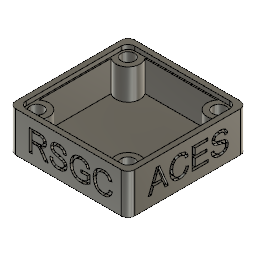
MyLEDTesterCase (Autodesk Fusion 360 design; units mm, degrees)
Autodesk Fusion 360 part; units mm, degrees
note: some values were not read from the file. Chosen so that the rebuilt part matches the saved one: that a step has no effect; the layout of a text. Set by a fixed rule: which sketch regions a step uses.
sketch "PCB" plane through (0, 0, 0) normal (0, 0, 1) x (1, 0, 0)
  line L0 (0, 0) -> (40, 0)
  line L1 (40, 0) -> (40, 40)
  line L2 (40, 40) -> (0, 40)
  line L3 (0, 40) -> (0, 0)
  line L4 (-0.25, -0.25) -> (40.25, -0.25)
  line L5 (40.25, -0.25) -> (40.25, 40.25)
  line L6 (40.25, 40.25) -> (-0.25, 40.25)
  line L7 (-0.25, 40.25) -> (-0.25, -0.25)
  line L8 (39.75, 0.25) -> (39.75, 39.75)
  line L9 (39.75, 39.75) -> (0.25, 39.75)
  line L10 (0.25, 39.75) -> (0.25, 0.25)
  line L11 (0.25, 0.25) -> (39.75, 0.25)
  line L12 (42.25, 42.25) -> (-2.25, 42.25)
  line L13 (-2.25, 42.25) -> (-2.25, -2.25)
  line L14 (-2.25, -2.25) -> (42.25, -2.25)
  line L15 (42.25, -2.25) -> (42.25, 42.25)
  dimension "d7" = 40
  dimension "d8" = 40
  dimension "d30" = 0.25
  dimension "d32" = 2.25
  constraint horizontal L0
  constraint vertical L1
  constraint horizontal L2
  constraint vertical L3
  constraint coincident L0.start L3.end
  measures "d7" distance of L0.start L0.end
  measures "d8" distance of L0.start L2.end
sketch "Piers" plane through (0, 0, 0) normal (0, 0, 1) x (1, 0, 0)
  line L0 (40, 40) -> (0, 40)
  circle A0 centre (3, 37) radius 4.5
  circle A1 centre (3, 37) radius 2.5
  line L1 (0, 40) -> (0, 0)
  line L2 (0, 0) -> (40, 0)
  circle A2 centre (3, 3) radius 4.5
  circle A3 centre (3, 3) radius 2.5
  line L3 (40, 0) -> (40, 40)
  circle A4 centre (37, 37) radius 4.5
  circle A5 centre (37, 37) radius 2.5
  circle A6 centre (37, 3) radius 4.5
  circle A7 centre (37, 3) radius 2.5
  point P0 (3, 37)
  point P1 (0, 40)
  point P2 (3, 3)
  point P3 (37, 37)
  point P4 (37, 3)
  point P5 (37, 3)
  dimension "d10" = 3
  dimension "d11" = 3
  dimension "d13" = 9
  dimension "d15" = 5
  dimension "d16" = 3
  dimension "d17" = 3
  dimension "d18" = 9
  dimension "d19" = 5
  dimension "d20" = 3
  dimension "d21" = 3
  dimension "d22" = 9
  dimension "d23" = 5
  dimension "d24" = 3
  dimension "d25" = 3
  dimension "d26" = 9
  dimension "d27" = 5
  constraint coincident P0 A0.centre
  constraint coincident P2 A2.centre
  constraint coincident P3 A4.centre
  constraint coincident P5 P4
  constraint concentric A6 A7
  measures "d10" horizontal distance of P0 L0.end
  measures "d11" distance of P0 L0
  measures "d13" diameter of A0
  measures "d15" diameter of A1
  measures "d16" distance of P2 L1
  measures "d17" distance of P2 L2
  measures "d18" diameter of A2
  measures "d19" diameter of A3
  measures "d20" distance of P3 L3
  measures "d21" distance of L0 P3
  measures "d22" diameter of A4
  measures "d23" diameter of A5
  measures "d24" distance of L3 P5
  measures "d25" distance of L2 P5
  measures "d26" diameter of A6
  measures "d27" diameter of A7
extrude "Extrude1" add sketch "Piers" along normal blind 13.4 contours L0 L3 A4 | L0 L3 A4 makes body 1
extrude "Extrude2" add sketch "Piers" along normal blind 6 contours A5 bodies 1
extrude "Extrude3" add sketch "Piers" along normal blind 6 separate body contours A7 makes body 2
extrude "Extrude4" add sketch "Piers" along normal blind 13.4 contours L2 L3 A6 | L2 L3 A6 bodies 2
extrude "Extrude5" add sketch "Piers" along normal blind 6 separate body contours A3 makes body 3
extrude "Extrude6" add sketch "Piers" along normal blind 13.4 contours L1 L2 A2 | L1 L2 A2 bodies 3
extrude "Extrude7" add sketch "Piers" along normal blind 6 separate body contours A1 makes body 4
extrude "Extrude8" add sketch "Piers" along normal blind 13.4 contours L0 A0 L1 | L0 A0 L1 bodies 4
extrude "Extrude9" cut sketch "PCB" along normal blind 2 contours L8 L9 L10 L11 bodies 1 2 3 4
extrude "Extrude10" add sketch "PCB" along normal blind 2 contours L8 L9 L10 L11 bodies 1 2 3 4
extrude "Extrude11" add sketch "PCB" along normal blind 13.4 contours L0 L1 L2 L3 bodies 1
extrude "Extrude12" add sketch "PCB" along normal blind 13.4 contours L4 L5 L6 L7 bodies 1
extrude "Extrude13" add sketch "PCB" along normal blind 15 contours L12 L13 L14 L15 bodies 1
fillet "Fillet1" radius 2.54 4 edges at (42.25, -2.25, 7.5) (-2.25, -2.25, 7.5) (42.25, 42.25, 7.5) (-2.25, 42.25, 7.5) on bodies 1
fillet "Fillet2" radius 2.54 1 edges at (40.25, -0.25, 14.2) on bodies 1
fillet "Fillet3" radius 2.54 1 edges at (-0.25, 40.25, 14.2) on bodies 1
fillet "Fillet4" radius 2.54 1 edges at (-0.25, -0.25, 14.2) on bodies 1
fillet "Fillet5" radius 2.54 1 edges at (40.25, 40.25, 14.2) on bodies 1
extrude "Extrude15" [no effect]
sketch "Sketch14" plane through (0, -2.25, 0) normal (0, -1, 0) x (1, 0, 0)
  line L0 (0.29, 15) -> (0.29, 0)
  line L1 (0.29, 0) -> (39.71, 0)
  line L2 (39.71, 0) -> (39.71, 15)
  line L3 (39.71, 15) -> (0.29, 15)
  line L4 (3.6628, 2.2796) -> (38.1217, 2.2796) construction
  line L5 (38.1217, 2.2796) -> (38.1217, 12.6948) construction
  line L6 (38.1217, 12.6948) -> (3.6628, 12.6948) construction
  line L7 (3.6628, 12.6948) -> (3.6628, 2.2796) construction
  line L8 (20, 15) -> (20, 0) construction
  line L9 (0.29, 7.5) -> (39.71, 7.5) construction
  dimension "d84" = 8
  text T0 "RSGC" font "Arial" height 8 align centre middle in box 34.4588 x 10.4152 at (3.6628, 2.2796) x (1, 0) y (0, 1) spacing 1
  constraint midpoint L3 L8.start
  constraint midpoint L1 L8.end
  constraint midpoint L0 L9.start
  constraint midpoint L2 L9.end
extrude "Extrude16" cut sketch "Sketch14" against normal blind 1 text T0 bodies 1
sketch "Sketch15" plane through (42.25, 0, 0) normal (1, 0, 0) x (0, 1, 0)
  line L0 (39.71, 0) -> (39.71, 15)
  line L1 (39.71, 15) -> (0.29, 15)
  line L2 (0.29, 15) -> (0.29, 0)
  line L3 (0.29, 0) -> (39.71, 0)
  line L4 (2.6602, 2.4104) -> (37.8312, 2.4104) construction
  line L5 (37.8312, 2.4104) -> (37.8312, 13.0108) construction
  line L6 (37.8312, 13.0108) -> (2.6602, 13.0108) construction
  line L7 (2.6602, 13.0108) -> (2.6602, 2.4104) construction
  dimension "d87" = 8
  text T0 "ACES" font "Arial" height 8 align centre middle in box 35.171 x 10.6004 at (2.6602, 2.4104) x (1, 0) y (0, 1) spacing 1
extrude "Extrude17" cut sketch "Sketch15" against normal blind 1 text T0 bodies 1
sketch "Sketch16" plane through (0, 42.25, 0) normal (0, 1, 0) x (-1, 0, 0)
  line L0 (-0.29, 0) -> (-0.29, 15)
  line L1 (-0.29, 15) -> (-39.71, 15)
  line L2 (-39.71, 15) -> (-39.71, 0)
  line L3 (-39.71, 0) -> (-0.29, 0)
  line L4 (-38.4676, 1.9614) -> (-1.8104, 1.9614) construction
  line L5 (-1.8104, 1.9614) -> (-1.8104, 13.8308) construction
  line L6 (-1.8104, 13.8308) -> (-38.4676, 13.8308) construction
  line L7 (-38.4676, 13.8308) -> (-38.4676, 1.9614) construction
  dimension "d90" = 4
  text T0 "LED Tester" font "Arial" height 4 align centre middle in box 36.6572 x 11.8695 at (-38.4676, 1.9614) x (1, 0) y (0, 1) spacing 1 kerned
extrude "Extrude18" cut sketch "Sketch16" against normal blind 1 text T0 bodies 1
sketch "Revised_ACESLogoOutline-01" plane through (-2.25, 14.4902, 3.4358) normal (-1, 0, 0) x (0, -1, 0)
  line L0 (5.7875, 4.2153) -> (5.7875, 5.4361)
  spline S0 degree 3 poles (5.7875, 5.4361) (5.7875, 5.4722) (5.7722, 5.5181) (5.8194, 5.5347) knots 1 1 1 1 2 2 2 2
  arc A0 (5.8194, 5.5347) -> (5.9472, 5.5069) centre (5.8593, 5.4104) cw
  arc A1 (5.9472, 5.5069) -> (6.075, 5.3583) centre (5.2544, 4.782) cw
  spline S1 degree 3 poles (6.075, 5.3583) (6.3458, 5.0319) (6.6208, 4.7069) (6.8833, 4.3736) knots 4 4 4 4 5 5 5 5
  spline S2 degree 3 poles (6.8833, 4.3736) (7.1224, 4.1027) (7.0966, 3.6893) (6.8257, 3.4503) (6.6775, 3.3195) (6.4782, 3.2628) (6.2833, 3.2958) knots 5 5 5 5 6 6 6 7 7 7 7
  spline S3 degree 3 poles (6.2833, 3.2958) (6.2083, 3.3069) (6.1361, 3.3194) (6.0625, 3.3375) knots 7 7 7 7 8 8 8 8
  spline S4 degree 3 poles (6.0625, 3.3375) (6.0514, 3.3375) (6.0417, 3.3528) (6.0194, 3.3222) (6.0306, 3.3167) (6.0306, 3.3042) knots 8 8 8 8 9 9 10 10 10 10
  arc A2 (6.0306, 3.3042) -> (6.1597, 3.0264) centre (7.2606, 3.7072) ccw
  spline S5 degree 3 poles (6.1597, 3.0264) (6.1819, 2.9875) (6.2264, 2.9514) (6.1736, 2.8542) (6.1181, 2.875) (6.075, 2.8736) knots 11 11 11 11 12 12 13 13 13 13
  line L1 (6.075, 2.8736) -> (5.8667, 2.8736)
  spline S6 degree 3 poles (5.8667, 2.8736) (5.7972, 2.8736) (5.7861, 2.8875) (5.7861, 2.9528) knots 14 14 14 14 15 15 15 15
  line L2 (5.7861, 2.9528) -> (5.7875, 4.2153)
  arc A3 (2.1694, 1.7181) -> (1.7806, 1.6611) centre (1.7638, 3.1319) cw
  ellipse E0 centre (1.7853, 2.2986) end of major axis (2.3346, 1.9689) minor radius 0.6364 (1.225, 1.9944) -> (1.7806, 1.6611) ccw
  arc A4 (1.225, 1.9944) -> (1.1681, 2.4625) centre (1.7577, 2.2967) cw
  ellipse E1 centre (1.2433, 2.4488) end of major axis (1.3045, 2.4956) minor radius 0.076 (1.25, 2.525) -> (1.1681, 2.4625) ccw
  line L3 (1.25, 2.525) -> (2.3208, 2.525)
  spline S7 degree 3 poles (2.3208, 2.525) (2.3917, 2.525) (2.4042, 2.5097) (2.4042, 2.4361) knots 5 5 5 5 6 6 6 6
  line L4 (2.4042, 2.4361) -> (2.4042, 1.3375)
  spline S8 degree 3 poles (2.4042, 1.3375) (2.4042, 1.2778) (2.3847, 1.2556) (2.3236, 1.2556) knots 7 7 7 7 8 8 8 8
  line L5 (2.3236, 1.2556) -> (2.0667, 1.2556)
  arc A5 (2.0667, 1.2556) -> (1.9889, 1.2875) centre (2.0526, 1.3321) cw
  spline S9 degree 3 poles (1.9889, 1.2875) (1.9694, 1.3194) (1.9889, 1.3403) (2.0042, 1.3639) knots 10 10 10 10 11 11 11 11
  arc A6 (2.0042, 1.3639) -> (2.1694, 1.7181) centre (1.0484, 2.0256) ccw
  line L6 (5.7986, 6.5347) -> (5.7986, 7.0903)
  spline S10 degree 3 poles (5.7986, 7.0903) (5.7986, 7.1639) (5.8333, 7.1944) (5.9153, 7.1708) knots 1 1 1 1 2 2 2 2
  arc A7 (5.9153, 7.1708) -> (5.9972, 7.1153) centre (5.8669, 7.0113) cw
  line L7 (5.9972, 7.1153) -> (6.4139, 6.6042)
  line L8 (6.4139, 6.6042) -> (6.8778, 6.0486)
  arc A8 (6.8778, 6.0486) -> (6.9139, 6.0014) centre (6.7098, 5.8827) cw
  ellipse E2 centre (6.8722, 5.973) end of major axis (6.8826, 6.0227) minor radius 0.05 (6.899, 5.9303) -> (6.9139, 6.0014) ccw
  ellipse E3 centre (6.8619, 5.9709) end of major axis (6.9184, 5.9567) minor radius 0.0493 (6.8972, 5.9292) -> (6.899, 5.9303) ccw
  ellipse E4 centre (6.8672, 5.979) end of major axis (6.9228, 5.9965) minor radius 0.0582 (6.8681, 5.9208) -> (6.8972, 5.9292) ccw
  line L9 (6.8681, 5.9208) -> (5.8514, 5.9208)
  spline S11 degree 3 poles (5.8514, 5.9208) (5.8014, 5.9208) (5.7972, 5.9556) (5.7972, 5.9944) knots 10 10 10 10 11 11 11 11
  line L10 (5.7972, 5.9944) -> (5.7972, 6.5347)
  line L11 (5.7972, 6.5347) -> (5.7986, 6.5347)
  line L12 (4.0931, 7.5153) -> (3.6764, 7.5153)
  spline S12 degree 3 poles (3.6764, 7.5153) (3.6444, 7.5153) (3.6167, 7.5153) (3.5861, 7.5875) (3.6014, 7.6042) (3.6236, 7.6264) knots 1 1 1 1 2 2 3 3 3 3
  line L13 (3.6236, 7.6264) -> (3.9625, 8.0431)
  spline S13 degree 3 poles (3.9625, 8.0431) (4.0285, 8.1166) (4.1416, 8.1228) (4.2153, 8.0569) knots 4 4 4 4 5 5 5 5
  ellipse E5 centre (4.1301, 7.958) end of major axis (4.2598, 7.9426) minor radius 0.1305 (4.2292, 8.0431) -> (4.2153, 8.0569) ccw
  spline S14 degree 3 poles (4.2292, 8.0431) (4.3472, 7.9042) (4.4597, 7.7653) (4.575, 7.6194) knots 6 6 6 6 7 7 7 7
  spline S15 degree 3 poles (4.575, 7.6194) (4.5931, 7.5986) (4.6125, 7.5778) (4.5944, 7.5458) knots 7 7 7 7 8 8 8 8
  arc A9 (4.5944, 7.5458) -> (4.5194, 7.5111) centre (4.5321, 7.5822) cw
  line L14 (4.5194, 7.5111) -> (4.0931, 7.5153)
  line L15 (4.1, 0.3319) -> (3.7958, 0.3319)
  arc A10 (3.7958, 0.3319) -> (3.7347, 0.3597) centre (3.7857, 0.3908) cw
  arc A11 (3.7347, 0.3597) -> (3.7444, 0.4319) centre (3.7965, 0.3882) cw
  arc A12 (3.7444, 0.4319) -> (3.9139, 0.7847) centre (2.8356, 1.0855) ccw
  line L16 (3.9139, 0.7847) -> (3.9139, 0.7958)
  spline S16 degree 3 poles (3.9139, 0.7958) (3.9417, 0.9347) (3.9417, 0.9347) (4.0778, 0.9347) knots 5 5 5 5 6 6 6 6
  line L17 (4.0778, 0.9347) -> (4.1847, 0.9347)
  spline S17 degree 3 poles (4.1847, 0.9347) (4.2192, 0.9406) (4.252, 0.9177) (4.2583, 0.8833) knots 7 7 7 7 8 8 8 8
  ellipse E6 centre (4.2409, 0.8792) end of major axis (4.2409, 0.8972) minor radius 0.0179 (4.2583, 0.875) -> (4.2583, 0.8833) ccw
  arc A13 (4.2583, 0.875) -> (4.4444, 0.4444) centre (5.174, 1.0153) ccw
  arc A14 (4.4444, 0.4444) -> (4.4597, 0.3556) centre (4.3719, 0.3862) cw
  spline S18 degree 3 poles (4.4597, 0.3556) (4.4472, 0.3264) (4.4139, 0.3319) (4.3861, 0.3319) knots 11 11 11 11 12 12 12 12
  line L18 (4.3861, 0.3319) -> (4.1, 0.3319)
  line L19 (5.0403, 5.9069) -> (4.5167, 5.9069)
  spline S19 degree 3 poles (4.5167, 5.9069) (4.3181, 5.9069) (4.1181, 5.8972) (3.9194, 5.9069) knots 1 1 1 1 2 2 2 2
  line L20 (3.9194, 5.9069) -> (3.1083, 5.9069)
  arc A15 (3.1083, 5.9069) -> (3.0403, 5.9417) centre (3.1014, 5.9774) cw
  arc A16 (3.0403, 5.9417) -> (3.0556, 6.0125) centre (3.0943, 5.9671) cw
  arc A17 (3.0556, 6.0125) -> (3.95, 7.0986) centre (198.9136, -154.3711) cw
  spline S20 degree 3 poles (3.95, 7.0986) (4.0042, 7.1801) (4.1141, 7.2025) (4.1958, 7.1486) knots 6 6 6 6 7 7 7 7
  arc A18 (4.1958, 7.1486) -> (4.2514, 7.0903) centre (4.1024, 7.004) cw
  spline S21 degree 3 poles (4.2514, 7.0903) (4.375, 6.9361) (4.5042, 6.7861) (4.6306, 6.6333) knots 8 8 8 8 9 9 9 9
  line L21 (4.6306, 6.6333) -> (5.0472, 6.1236)
  spline S22 degree 3 poles (5.0472, 6.1236) (5.0778, 6.0861) (5.1069, 6.0486) (5.1389, 6.0139) knots 10 10 10 10 11 11 11 11
  arc A19 (5.1389, 6.0139) -> (5.1542, 5.9444) centre (5.1014, 5.9692) cw
  arc A20 (5.1542, 5.9444) -> (5.0875, 5.9083) centre (5.0989, 5.967) cw
  ellipse E7 centre (5.0679, 5.7711) end of major axis (5.2065, 5.7774) minor radius 0.1386 (5.0875, 5.9083) -> (5.0403, 5.9069) ccw
  spline S23 degree 3 poles (2.1708, 3.3514) (2.0806, 3.3292) (1.9944, 3.3111) (1.9083, 3.2972) knots 0 0 0 0 1 1 1 1
  spline S24 degree 3 poles (1.9083, 3.2972) (1.5517, 3.2392) (1.2156, 3.4812) (1.1576, 3.8378) (1.1271, 4.0253) (1.1795, 4.2168) (1.3014, 4.3625) knots 1 1 1 1 2 2 2 3 3 3 3
  spline S25 degree 3 poles (1.3014, 4.3625) (1.4722, 4.5833) (1.6542, 4.7944) (1.8292, 5.0097) knots 3 3 3 3 4 4 4 4
  line L22 (1.8292, 5.0097) -> (2.2069, 5.4708)
  arc A21 (2.2069, 5.4708) -> (2.3458, 5.5403) centre (2.3416, 5.3751) cw
  spline S26 degree 3 poles (2.3458, 5.5403) (2.3803, 5.5418) (2.4095, 5.5152) (2.4111, 5.4807) knots 6 6 6 6 7 7 7 7
  line L23 (2.4111, 5.4807) -> (2.4111, 5.4806)
  line L24 (2.4111, 5.4806) -> (2.4111, 2.9583)
  spline S27 degree 3 poles (2.4111, 2.9583) (2.4189, 2.9227) (2.3966, 2.8874) (2.3611, 2.8792) knots 9 9 9 9 10 10 10 10
  line L25 (2.3611, 2.8792) -> (2.0639, 2.8792)
  arc A22 (2.0639, 2.8792) -> (1.9889, 2.9167) centre (2.0542, 2.9535) cw
  spline S28 degree 3 poles (1.9889, 2.9167) (1.9708, 2.9431) (1.9889, 2.9653) (2.0028, 2.9861) knots 12 12 12 12 13 13 13 13
  arc A23 (2.0028, 2.9861) -> (2.1708, 3.3514) centre (0.989, 3.6738) ccw
  arc A24 (3.9153, 3.3514) -> (3.5181, 3.2889) centre (3.4967, 4.7179) cw
  spline S29 degree 3 poles (3.5181, 3.2889) (3.2021, 3.3071) (2.9433, 3.5463) (2.9, 3.8597) knots 1 1 1 1 2 2 2 2
  arc A25 (2.9, 3.8597) -> (3.0792, 4.4069) centre (3.6477, 3.9178) cw
  spline S30 degree 3 poles (3.0792, 4.4069) (3.3681, 4.7611) (3.6611, 5.1125) (3.95, 5.4681) knots 3 3 3 3 4 4 4 4
  spline S31 degree 3 poles (3.95, 5.4681) (4.013, 5.55) (4.1304, 5.5655) (4.2125, 5.5028) knots 4 4 4 4 5 5 5 5
  ellipse E8 centre (4.1155, 5.3711) end of major axis (4.2313, 5.2553) minor radius 0.1636 (4.2472, 5.4681) -> (4.2125, 5.5028) ccw
  spline S32 degree 3 poles (4.2472, 5.4681) (4.4208, 5.2472) (4.6056, 5.0375) (4.7833, 4.8208) knots 6 6 6 6 7 7 7 7
  arc A26 (4.7833, 4.8208) -> (5.1833, 4.3236) centre (0.7095, 1.1341) cw
  spline S33 degree 3 poles (5.1833, 4.3236) (5.3917, 4.0324) (5.3253, 3.6274) (5.0347, 3.4181) knots 8 8 8 8 9 9 9 9
  arc A27 (5.0347, 3.4181) -> (4.8042, 3.3139) centre (4.6499, 3.9625) cw
  arc A28 (4.8042, 3.3139) -> (4.3583, 3.3361) centre (4.6263, 4.2287) cw
  spline S34 degree 3 poles (4.3583, 3.3361) (4.3333, 3.3361) (4.3, 3.3681) (4.2667, 3.3264) (4.2931, 3.2972) (4.3014, 3.2722) knots 11 11 11 11 12 12 13 13 13 13
  arc A29 (4.3014, 3.2722) -> (4.4444, 3.0181) centre (5.7116, 3.8986) ccw
  spline S35 degree 3 poles (4.4444, 3.0181) (4.4625, 2.9903) (4.4861, 2.9611) (4.4444, 2.8889) (4.4097, 2.8958) (4.375, 2.8958) knots 14 14 14 14 15 15 16 16 16 16
  line L26 (4.375, 2.8958) -> (3.8194, 2.8958)
  arc A30 (3.8194, 2.8958) -> (3.7486, 2.9278) centre (3.8124, 2.9747) cw
  spline S36 degree 3 poles (3.7486, 2.9278) (3.7292, 2.9569) (3.7486, 2.9806) (3.7597, 3.0042) knots 18 18 18 18 19 19 19 19
  arc A31 (3.7597, 3.0042) -> (3.9153, 3.3514) centre (2.8462, 3.6219) ccw
  arc A32 (4.2764, 1.7194) -> (4.4292, 1.3819) centre (5.3765, 2.0141) ccw
  ellipse E9 centre (4.1267, 1.1484) end of major axis (4.4904, 1.2657) minor radius 0.382 (4.4556, 1.3431) -> (4.4292, 1.3819) ccw
  ellipse E10 centre (4.4083, 1.3132) end of major axis (4.4218, 1.3679) minor radius 0.0554 (4.4364, 1.2648) -> (4.4556, 1.3431) ccw
  line L27 (4.4364, 1.2648) -> (4.4347, 1.2639)
  arc A33 (4.4347, 1.2639) -> (4.4014, 1.2556) centre (4.407, 1.3038) cw
  line L28 (4.4014, 1.2556) -> (3.7917, 1.2556)
  spline S37 degree 3 poles (3.7917, 1.2556) (3.7347, 1.2556) (3.7125, 1.3) (3.7431, 1.35) knots 6 6 6 6 7 7 7 7
  arc A34 (3.7431, 1.35) -> (3.8986, 1.6542) centre (2.5289, 2.1628) ccw
  spline S38 degree 3 poles (3.8986, 1.6542) (3.9056, 1.6736) (3.9181, 1.6958) (3.8792, 1.7236) (3.8667, 1.7097) (3.85, 1.7014) knots 8 8 8 8 9 9 10 10 10 10
  arc A35 (3.85, 1.7014) -> (3.2861, 1.7097) centre (3.5805, 2.5499) cw
  spline S39 degree 3 poles (3.2861, 1.7097) (3.0523, 1.8099) (2.8986, 2.0374) (2.8931, 2.2917) knots 11 11 11 11 12 12 12 12
  arc A36 (2.8931, 2.2917) -> (2.9167, 2.4833) centre (3.6347, 2.2976) cw
  ellipse E11 centre (2.9773, 2.4738) end of major axis (3.0267, 2.5111) minor radius 0.061 (2.9847, 2.5347) -> (2.9167, 2.4833) ccw
  line L29 (2.9847, 2.5347) -> (5.175, 2.5347)
  spline S40 degree 3 poles (5.175, 2.5347) (5.2375, 2.5347) (5.2653, 2.5139) (5.2778, 2.4569) knots 15 15 15 15 16 16 16 16
  spline S41 degree 3 poles (5.2778, 2.4569) (5.3641, 2.114) (5.1561, 1.766) (4.8132, 1.6797) knots 16 16 16 16 17 17 17 17
  line L30 (4.8132, 1.6797) -> (4.8111, 1.6792)
  line L31 (4.8111, 1.6792) -> (4.7903, 1.6792)
  arc A37 (4.7903, 1.6792) -> (4.2764, 1.7194) centre (4.6137, 2.7241) cw
  spline S42 degree 3 poles (2.4, 6.6764) (2.4125, 6.5181) (2.3931, 6.3306) (2.4083, 6.1444) knots 0 0 0 0 1 1 1 1
  line L32 (2.4083, 6.1444) -> (2.4083, 5.9681)
  ellipse E12 centre (2.35, 5.9627) end of major axis (2.3886, 6.0074) minor radius 0.0581 (2.3531, 5.9042) -> (2.4083, 5.9681) ccw
  line L33 (2.3531, 5.9042) -> (2.3528, 5.9042)
  line L34 (2.3528, 5.9042) -> (1.7194, 5.9042)
  line L35 (1.7194, 5.9042) -> (1.3444, 5.9042)
  ellipse E13 centre (1.3377, 5.9569) end of major axis (1.3795, 5.9233) minor radius 0.0527 (1.2848, 5.9522) -> (1.3444, 5.9042) ccw
  line L36 (1.2848, 5.9522) -> (1.2847, 5.9528)
  arc A38 (1.2847, 5.9528) -> (1.3028, 5.9986) centre (1.3415, 5.9569) cw
  spline S43 degree 3 poles (1.3028, 5.9986) (1.4417, 6.1667) (1.5806, 6.3347) (1.7194, 6.5) knots 9 9 9 9 10 10 10 10
  line L37 (1.7194, 6.5) -> (2.0833, 6.9681)
  spline S44 degree 3 poles (2.0833, 6.9681) (2.1236, 7.0181) (2.1653, 7.0694) (2.2069, 7.1181) knots 11 11 11 11 12 12 12 12
  arc A39 (2.2069, 7.1181) -> (2.3264, 7.1736) centre (2.3325, 7.0043) cw
  spline S45 degree 3 poles (2.3264, 7.1736) (2.3599, 7.1778) (2.3904, 7.154) (2.3946, 7.1206) (2.3953, 7.1151) (2.3952, 7.1096) (2.3944, 7.1042) knots 13 13 13 13 14 14 14 15 15 15 15
  spline S46 degree 3 poles (2.3944, 7.1042) (2.3986, 6.9708) (2.4, 6.8375) (2.4, 6.6764) knots 15 15 15 15 16 16 16 16
  line L38 (7.3931, 3.9986) -> (7.3931, 4.5778)
  spline S47 degree 3 poles (7.3931, 4.5778) (7.3931, 4.6097) (7.3931, 4.6403) (7.4278, 4.6528) knots 1 1 1 1 2 2 2 2
  arc A40 (7.4278, 4.6528) -> (7.5028, 4.6319) centre (7.4532, 4.5987) cw
  spline S48 degree 3 poles (7.5028, 4.6319) (7.5833, 4.525) (7.6819, 4.4306) (7.7528, 4.3153) knots 3 3 3 3 4 4 4 4
  spline S49 degree 3 poles (7.7528, 4.3153) (7.9086, 4.0935) (7.9119, 3.7988) (7.7611, 3.5736) knots 4 4 4 4 5 5 5 5
  arc A41 (7.7611, 3.5736) -> (7.5, 3.3542) centre (7.1974, 3.9792) cw
  ellipse E14 centre (7.6408, 3.7197) end of major axis (7.8605, 4.0943) minor radius 0.1394 (7.3903, 3.425) -> (7.5, 3.3542) ccw
  line L39 (7.3903, 3.425) -> (7.3903, 3.9986)
  line L40 (7.3903, 3.9986) -> (7.3931, 3.9986)
  line L41 (0.7958, 3.9903) -> (0.7958, 3.4208)
  ellipse E15 centre (0.2764, 4.168) end of major axis (-0.215, 4.9919) minor radius 0.1958 (0.6903, 3.3542) -> (0.7958, 3.4208) ccw
  arc A42 (0.6903, 3.3542) -> (0.3306, 3.8167) centre (0.9573, 3.933) cw
  arc A43 (0.3306, 3.8167) -> (0.4875, 4.3833) centre (1.0153, 3.9321) cw
  spline S50 degree 3 poles (0.4875, 4.3833) (0.5556, 4.4681) (0.6222, 4.5458) (0.6944, 4.6347) knots 4 4 4 4 5 5 5 5
  arc A44 (0.6944, 4.6347) -> (0.7639, 4.6542) centre (0.7415, 4.6003) cw
  spline S51 degree 3 poles (0.7639, 4.6542) (0.7944, 4.6431) (0.8014, 4.6194) (0.8014, 4.5889) knots 6 6 6 6 7 7 7 7
  spline S52 degree 3 poles (0.8014, 4.5889) (0.7944, 4.3903) (0.7958, 4.1931) (0.7958, 3.9903) knots 7 7 7 7 8 8 8 8
  arc A45 (6.0403, 1.7167) -> (6.2, 1.3778) centre (7.2495, 2.0795) ccw
  spline S53 degree 3 poles (6.2, 1.3778) (6.2167, 1.3514) (6.2361, 1.3264) (6.2, 1.2569) (6.1681, 1.2653) (6.1403, 1.2653) knots 1 1 1 1 2 2 3 3 3 3
  line L42 (6.1403, 1.2653) -> (5.8736, 1.2653)
  spline S54 degree 3 poles (5.8736, 1.2653) (5.8208, 1.2653) (5.8, 1.2875) (5.8, 1.3403) knots 4 4 4 4 5 5 5 5
  line L43 (5.8, 1.3403) -> (5.8, 2.4625)
  spline S55 degree 3 poles (5.8, 2.4625) (5.8, 2.5139) (5.8222, 2.5403) (5.8736, 2.5403) knots 6 6 6 6 7 7 7 7
  line L44 (5.8736, 2.5403) -> (6.9625, 2.5403)
  ellipse E16 centre (6.972, 2.4782) end of major axis (7.0242, 2.4424) minor radius 0.0624 (7.0333, 2.4917) -> (6.9625, 2.5403) ccw
  spline S56 degree 3 poles (7.0333, 2.4917) (7.1304, 2.1484) (6.9308, 1.7915) (6.5876, 1.6945) knots 9 9 9 9 10 10 10 10
  line L45 (6.5876, 1.6945) -> (6.5875, 1.6944)
  arc A46 (6.5875, 1.6944) -> (6.4972, 1.6764) centre (6.4065, 2.3649) cw
  arc A47 (6.4972, 1.6764) -> (6.0806, 1.7236) centre (6.4118, 2.7842) cw
  line L46 (6.0806, 1.7236) -> (6.0569, 1.7236)
  line L47 (6.0569, 1.7236) -> (6.0403, 1.7167)
extrude "Extrude19" cut sketch "Revised_ACESLogoOutline-01" against normal blind 1 bodies 1
equation "pcbWidth = 40 mm"
equation "pcbHeight = 40 mm"
equation "d7 = pcbWidth"
equation "d8 = pcbHeight"
equation "pierCornerOffset = 3 mm"
equation "d10 = pierCornerOffset"
equation "d11 = pierCornerOffset"
equation "pierOuterDiameter = 9 mm"
equation "d13 = pierOuterDiameter"
equation "pierInnerDiameter = 5 mm"
equation "d15 = pierInnerDiameter"
equation "d16 = pierCornerOffset"
equation "d17 = pierCornerOffset"
equation "d18 = pierOuterDiameter"
equation "d19 = pierInnerDiameter"
equation "d20 = pierCornerOffset"
equation "d21 = pierCornerOffset"
equation "d22 = pierOuterDiameter"
equation "d23 = pierInnerDiameter"
equation "d24 = pierCornerOffset"
equation "d25 = pierCornerOffset"
equation "d26 = pierOuterDiameter"
equation "d27 = pierInnerDiameter"
equation "pcbOffset = 0.25 mm"
equation "wallThickness = 2 mm"
equation "d30 = pcbOffset"
equation "d31 = -pcbOffset"
equation "d32 = pcbOffset + wallThickness"
equation "pierDepth = 7 mm"
equation "pcbThickness = 1.6 mm"
equation "caseHeight = 15 mm"
equation "pierHeight = caseHeight - pcbThickness"
equation "pierBaseHeight = caseHeight - pierDepth - wallThickness"
equation "d38 = pierHeight"
equation "d40 = pierBaseHeight"
equation "d42 = pierBaseHeight"
equation "d44 = pierHeight"
equation "d46 = pierBaseHeight"
equation "d48 = pierHeight"
equation "d50 = pierBaseHeight"
equation "d52 = pierHeight"
equation "d54 = wallThickness"
equation "d56 = wallThickness"
equation "d58 = pierHeight"
equation "d60 = pierHeight"
equation "d62 = caseHeight"
equation "filletRadius = 2.54 mm"
equation "d66 = filletRadius"
equation "d68 = filletRadius"
equation "d70 = filletRadius"
equation "d72 = filletRadius"
equation "d74 = filletRadius"
equation "textThickness = 1.5 mm"
equation "d82 = -textThickness"
